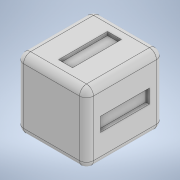
# Autodesk Inventor part: cube
Saved by Autodesk Inventor 2022 (Build 260153000, 153)
## iProperties
Created: 2023-03-11
Part Number: cube
Material: Типовые
Document SubType Name: Modeling
Designer: akapu
Density: 1 g/cm^3
Appearance: По умолчанию
Author: akapu
Autodesk Inventor part; units mm, degrees
ref_plane "YZ Plane" through (0, 0, 0) normal (1, 0, 0) x (0, 1, 0)
ref_plane "XZ Plane" through (0, 0, 0) normal (0, 1, 0) x (-1, 0, 0)
ref_plane "XY Plane" through (0, 0, 0) normal (0, 0, 1) x (1, 0, 0)
sketch "Эскиз1" plane through (0, 0, 0) normal (0, 1, 0) x (-1, 0, 0)
  line L0 (0, 0) -> (-10, 0)
  line L1 (-10, 0) -> (-10, -11)
  line L2 (-10, -11) -> (0, -11)
  line L3 (0, -11) -> (0, 0)
  dimension "d0" = 10
  dimension "d1" = 11
  constraints: 8 end point, 2 parallel, 1 horizontal, 1 perpendicular
  measures "d0" distance of L2.end L1.end
  measures "d1" distance of L1.end L0.end
extrude "Выдавливание1" add sketch "Эскиз1" along normal mid plane 10
sketch "Эскиз2" plane through (0, 0, 0) normal (0, 1, 0) x (-1, 0, 0)
  line L0 (0, -11) -> (0, 0) projected
  line L1 (0, -5.5) -> (-10, -5.5)
  line L2 (-10, 0) -> (-10, -11) projected
  line L3 (-1.5, -1.5) -> (-8.5, -1.5)
  line L4 (-8.5, -1.5) -> (-8.5, -9.5)
  line L5 (-8.5, -9.5) -> (-1.5, -9.5)
  line L6 (-1.5, -9.5) -> (-1.5, -1.5)
  line L7 (-1.5, -1.5) -> (-8.5, -9.5) construction
  line L8 (-8.5, -1.5) -> (-1.5, -9.5) construction
  point P0 (-5, -5.5)
  dimension "d4" = 7
  dimension "d5" = 8
  constraints: 14 end point, 5 midpoint, 2 parallel, 1 horizontal, 1 perpendicular
  measures "d4" distance of L5.end L4.end
  measures "d5" distance of L4.end L3.end
extrude "Выдавливание2" cut sketch "Эскиз2" along normal mid plane 7
fillet "Сопряжение1" radius 1 12 edges at (10, 5, -5.5) (5, -5, 0) (5, 5, 0) (0, 5, -5.5) (0, 0, 0) (0, -5, -5.5) (0, 0, -11) (10, 0, -11) (5, 5, -11) (5, -5, -11) (10, -5, -5.5) (10, 0, 0)
sketch "Эскиз3" plane through (0, -4, -1) normal (-1, 0, 0) x (0, 0, 1)
  line L0 (0, 0) -> (0, 8) projected
  line L1 (0, 4) -> (-9, 4)
  line L2 (-9, 0) -> (-9, 8) projected
  line L3 (-1, 5) -> (-8, 5)
  line L4 (-8, 5) -> (-8, 3)
  line L5 (-8, 3) -> (-1, 3)
  line L6 (-1, 3) -> (-1, 5)
  line L7 (-1, 5) -> (-8, 3) construction
  line L8 (-8, 5) -> (-1, 3) construction
  point P0 (1, 4)
  point P1 (-4.5, 4)
  constraints: 14 end point, 5 midpoint, 2 parallel, 1 horizontal, 1 perpendicular
sketch "Эскиз6" plane through (10, -4, -1) normal (1, 0, 0) x (0, 0, -1)
  line L0 (1, 3) -> (8, 3) projected
  line L1 (1, 5) -> (1, 3) projected
  line L2 (8, 5) -> (1, 5) projected
  line L3 (8, 3) -> (8, 5) projected
  point P0 (-1, 4)
sketch "Эскиз7" plane through (0, 5, 0) normal (0, 1, 0) x (1, 0, 0)
  line L0 (9, 1) -> (1, 1) projected
  line L1 (5, 1) -> (5, 10)
  line L2 (9, 10) -> (1, 10) projected
  line L3 (4, 2) -> (6, 2)
  line L4 (6, 2) -> (6, 9)
  line L5 (6, 9) -> (4, 9)
  line L6 (4, 9) -> (4, 2)
  line L7 (4, 2) -> (6, 9) construction
  line L8 (6, 2) -> (4, 9) construction
  point P0 (0, 0)
  point P1 (5, 5.5)
  constraints: 14 end point, 5 midpoint, 2 parallel, 1 horizontal, 1 perpendicular
sketch "Эскиз8" plane through (0, -5, 0) normal (0, -1, 0) x (1, 0, 0)
  line L0 (4, -9) -> (4, -2) projected
  line L1 (6, -9) -> (4, -9) projected
  line L2 (6, -2) -> (6, -9) projected
  line L3 (4, -2) -> (6, -2) projected
  point P0 (0, 0)
extrude "Выдавливание5" cut sketch "Эскиз7" against normal blind 0.5
extrude "Выдавливание6" cut sketch "Эскиз3" against normal blind 0.5
extrude "Выдавливание7" cut sketch "Эскиз8" against normal blind 0.5
extrude "Выдавливание8" cut sketch "Эскиз6" against normal blind 0.5
